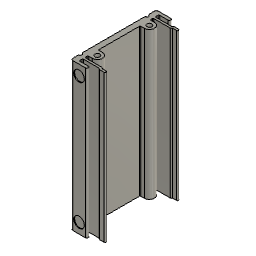
sidePanel_V2 v9 Fusion (Autodesk Fusion 360 design; units mm, degrees)
Autodesk Fusion 360 part; units mm, degrees
note: some values were not read from the file. Set by a fixed rule: which sketch regions a step uses.
sketch "Sketch1" plane through (0, 0, 0) normal (0, 0, 1) x (1, 0, 0)
  line L0 (36.0187, 148.7477) -> (36.0366, 148.794)
  line L1 (65.6521, 184) -> (76.1579, 184)
  line L2 (14.9996, 189) -> (14.9996, 194.9997)
  line L3 (-0.0194, 154.2247) -> (-0.0004, 154.2001)
  line L4 (-0.0302, 138.7537) -> (-0.0004, 138.7058)
  line L5 (-0.0004, 81.3672) -> (-0.0021, 81.3657)
  line L6 (15.3997, 143.0047) -> (15.3997, 102.5015)
  line L7 (-0.0004, 173.0047) -> (-0.0004, 102.5015)
  line L8 (2.0223, 183.0092) -> (1.9964, 183.0092)
  line L9 (1.9996, 175.0047) -> (2.0001, 175.0047)
  line L10 (4.0001, 177.0042) -> (4.0009, 181.0087)
  line L11 (0.0178, 200) -> (0.0178, 185.0092)
  arc A0 (0.0178, 185.0092) -> (2.0223, 183.0092) centre (2.0178, 185.0092) ccw
  arc A1 (4.0009, 181.0087) -> (1.9964, 183.0092) centre (2.0009, 181.0092) ccw
  line L12 (16.9996, 196.9997) -> (40, 196.9997)
  arc A2 (16.9996, 196.9997) -> (14.9996, 194.9997) centre (16.9996, 194.9997) ccw
  line L13 (16.9996, 187) -> (60, 187)
  arc A3 (14.9996, 189) -> (16.9996, 187) centre (16.9996, 189) ccw
  line L14 (63.5, 190) -> (76.1579, 190)
  line L15 (14.9996, 179.1547) -> (14.9996, 175.0047)
  arc A4 (16.9996, 181.1547) -> (14.9996, 179.1547) centre (16.9996, 179.1547) ccw
  line L16 (16.9996, 173.0047) -> (26.8487, 173.0047)
  arc A5 (14.9996, 175.0047) -> (16.9996, 173.0047) centre (16.9996, 175.0047) ccw
  arc A6 (2.0001, 175.0047) -> (4.0001, 177.0042) centre (2.0001, 177.0047) ccw
  arc A7 (1.9996, 175.0047) -> (-0.0004, 173.0047) centre (1.9996, 173.0047) ccw
  arc A8 (76.1579, 184) -> (76.1579, 190) centre (76.1579, 187) ccw
  line L17 (60, 187) -> (63.5, 190)
  line L18 (62.1079, 181.1547) -> (65.6521, 184)
  line L19 (17.3997, 145.0047) -> (27.1505, 145.0047)
  line L20 (27.4996, 145.0047) -> (27.5723, 145.0156)
  arc A9 (17.3997, 145.0047) -> (15.3997, 143.0047) centre (17.3997, 143.0047) ccw
  arc A10 (27.1505, 145.0047) -> (26.8487, 173.0047) centre (26.9996, 159.0047) ccw
  line L21 (-0.0004, 123.6359) -> (-0.0021, 123.6374)
  line L22 (5.0178, 205) -> (40, 205)
  arc A11 (5.0178, 205) -> (0.0178, 200) centre (5.0178, 200) ccw
  arc A12 (40, 196.9997) -> (40, 205) centre (40, 200.9999) ccw
  line L23 (16.9996, 181.1547) -> (62.1079, 181.1547)
  line L24 (27.4996, 29.9953) -> (27.5723, 29.9844)
  line L25 (16.9996, 1.9953) -> (26.8487, 1.9953)
  line L26 (16.9996, -12) -> (60, -12)
  line L27 (2.0223, -8.0092) -> (1.9964, -8.0092)
  line L28 (65.6521, -9) -> (76.1579, -9)
  arc A13 (1.9964, -8.0092) -> (4.0009, -6.0087) centre (2.0009, -6.0092) ccw
  line L29 (16.9996, -21.9997) -> (40, -21.9997)
  line L30 (1.9996, -0.0047) -> (2.0001, -0.0047)
  arc A14 (15.3997, 31.9953) -> (17.3997, 29.9953) centre (17.3997, 31.9953) ccw
  line L31 (36.0187, 26.2523) -> (36.0366, 26.206)
  arc A15 (0.0178, -25) -> (5.0178, -30) centre (5.0178, -25) ccw
  arc A16 (26.8487, 1.9953) -> (27.1505, 29.9953) centre (26.9996, 15.9953) ccw
  line L32 (4.0001, -2.0042) -> (4.0009, -6.0087)
  arc A17 (2.0223, -8.0092) -> (0.0178, -10.0092) centre (2.0178, -10.0092) ccw
  line L33 (16.9996, -6.1547) -> (62.1079, -6.1547)
  line L34 (5.0178, -30) -> (40, -30)
  arc A18 (16.9996, -12) -> (14.9996, -14) centre (16.9996, -14) ccw
  line L35 (14.9996, -4.1547) -> (14.9996, -0.0047)
  line L36 (63.5, -15) -> (76.1579, -15)
  arc A19 (40, -30) -> (40, -21.9997) centre (40, -25.9999) ccw
  arc A20 (76.1579, -15) -> (76.1579, -9) centre (76.1579, -12) ccw
  arc A21 (14.9996, -19.9997) -> (16.9996, -21.9997) centre (16.9996, -19.9997) ccw
  arc A22 (4.0001, -2.0042) -> (2.0001, -0.0047) centre (2.0001, -2.0047) ccw
  line L37 (-0.0004, 51.3641) -> (-0.0021, 51.3626)
  line L38 (17.3997, 29.9953) -> (27.1505, 29.9953)
  line L39 (60, -12) -> (63.5, -15)
  line L40 (-0.0004, 1.9953) -> (-0.0004, 72.4985)
  line L41 (0.0178, -25) -> (0.0178, -10.0092)
  line L42 (-0.0194, 20.7753) -> (-0.0004, 20.7999)
  line L43 (14.9996, -14) -> (14.9996, -19.9997)
  arc A23 (16.9996, 1.9953) -> (14.9996, -0.0047) centre (16.9996, -0.0047) ccw
  line L44 (62.1079, -6.1547) -> (65.6521, -9)
  line L45 (-0.0302, 36.2463) -> (-0.0004, 36.2942)
  arc A24 (-0.0004, 1.9953) -> (1.9996, -0.0047) centre (1.9996, 1.9953) ccw
  arc A25 (14.9996, -4.1547) -> (16.9996, -6.1547) centre (16.9996, -4.1547) ccw
  line L46 (15.3997, 31.9953) -> (15.3997, 72.4985)
  line L47 (-0.0004, 102.5015) -> (-0.0004, 72.4985)
  line L48 (15.3997, 102.5015) -> (15.3997, 72.4985)
  circle A26 centre (26.9996, 15.9953) radius 6.7755
  circle A27 centre (26.9996, 159.0047) radius 6.7755
  dimension "d8" = 2
  dimension "d9" = 2
  dimension "d11" = 2
  dimension "d13" = 2
  dimension "d18" = 2
  dimension "d19" = 2
  dimension "d27" = 2
  dimension "d28" = 2
  dimension "d34" = 3
  dimension "d35" = 2
  dimension "d40" = 5
  dimension "d41" = 4.0002
  dimension "d52" = 14.0008
  dimension "d55" = 235
  dimension "d57" = 14.0008
  dimension "d59" = 13.551
  dimension "d61" = 45.9953
  dimension "d62" = 45.9953
  dimension "d63" = 27
  dimension "d64" = 27
  dimension "d65" = 13.551
  constraint perpendicular L7 L9
  constraint tangent L11 A0
  constraint tangent L8 A0
  constraint tangent L8 A1
  constraint tangent L10 A1
  constraint horizontal L12
  constraint tangent L12 A2
  constraint tangent L2 A2
  constraint horizontal L13
  constraint tangent L2 A3
  constraint tangent L13 A3
  constraint horizontal L14
  constraint vertical L15
  constraint tangent L15 A4
  constraint horizontal L16
  constraint tangent L16 A5
  constraint tangent L15 A5
  constraint tangent L10 A6
  constraint tangent L9 A6
  constraint tangent L9 A7
  constraint tangent L7 A7
  constraint horizontal L1
  constraint tangent L14 A8
  constraint tangent L1 A8
  constraint horizontal L19
  constraint coincident L20.end A10
  constraint tangent L19 A9
  constraint tangent L6 A9
  constraint coincident L7 L3.end
  constraint coincident L7 L4.end
  constraint coincident L7 L5.start
  constraint vertical L7
  constraint vertical L6
  constraint horizontal L22
  constraint tangent L11 A11
  constraint tangent L22 A11
  constraint tangent L22 A12
  constraint tangent L12 A12
  constraint tangent A4 L23
  constraint horizontal L23
  constraint vertical L47
  constraint parallel L46 L48
  constraint concentric A16 A26
  constraint concentric A10 A27
  measures "d8" radius of A0
  measures "d9" radius of A1
  measures "d11" radius of A2
  measures "d13" radius of A3
  measures "d18" radius of A4
  measures "d19" radius of A5
  measures "d27" radius of A6
  measures "d28" radius of A7
  measures "d34" radius of A8
  measures "d35" radius of A9
  measures "d40" radius of A11
  measures "d41" radius of A12
  measures "d52" radius of A10
  measures "d55" distance of L22 L34
  measures "d57" radius of A16
  measures "d59" diameter of A26
  measures "d61" distance of A10.centre L22
  measures "d62" distance of A16.centre L34
  measures "d63" distance of L40 A16.centre
  measures "d64" distance of L7 A10.centre
  measures "d65" diameter of A27
extrude "Extrude4" add sketch "Sketch1" along normal blind 404.3634 contours L1 L2 L6 L7 L8 L10 L11 A0 A1 L12 A2 L13 A3 L14 L15 A4 L16 A5 A6 A7 A8 L17 L18 L19 A9 A10 L22 A11 A12 L23 L25 L26 L27 L28 A13 L29 A14 A15 A16 L32 A17 L33 L34 A18 L35 L36 A19 A20 A21 A22 L38 L39 L40 L41 L43 A23 L44 A24 A25 L46 L47 L48 | A26 | A27
sketch "Sketch2" plane through (0, 0, 404.3634) normal (0, 0, 1) x (-1, 0, 0)
  line L0 (-17.3997, -145.0047) -> (-27.1505, -145.0047)
  arc A0 (-27.1505, -145.0047) -> (-26.8487, -173.0047) centre (-26.9996, -159.0047) ccw
  line L1 (-26.8487, -173.0047) -> (-16.9996, -173.0047)
  arc A1 (-14.9996, -175.0047) -> (-16.9996, -173.0047) centre (-16.9996, -175.0047) ccw
  line L2 (-14.9996, -175.0047) -> (-14.9996, -179.1547)
  arc A2 (-16.9996, -181.1547) -> (-14.9996, -179.1547) centre (-16.9996, -179.1547) ccw
  line L3 (-16.9996, -181.1547) -> (-62.1079, -181.1547)
  line L4 (-62.1079, -181.1547) -> (-65.6521, -184)
  line L5 (-65.6521, -184) -> (-76.1579, -184)
  arc A3 (-76.1579, -184) -> (-76.1579, -190) centre (-76.1579, -187) ccw
  line L6 (-76.1579, -190) -> (-63.5, -190)
  line L7 (-63.5, -190) -> (-60, -187)
  line L8 (-60, -187) -> (-16.9996, -187)
  arc A4 (-14.9996, -189) -> (-16.9996, -187) centre (-16.9996, -189) ccw
  line L9 (-14.9996, -189) -> (-14.9996, -194.9997)
  arc A5 (-16.9996, -196.9997) -> (-14.9996, -194.9997) centre (-16.9996, -194.9997) ccw
  line L10 (-16.9996, -196.9997) -> (-40, -196.9997)
  arc A6 (-40, -196.9997) -> (-40, -205) centre (-40, -200.9999) ccw
  line L11 (-40, -205) -> (-5.0178, -205)
  arc A7 (-5.0178, -205) -> (-0.0178, -200) centre (-5.0178, -200) ccw
  line L12 (-0.0178, -200) -> (-0.0178, -185.0092)
  arc A8 (-0.0178, -185.0092) -> (-2.0223, -183.0092) centre (-2.0178, -185.0092) ccw
  line L13 (-2.0223, -183.0092) -> (-1.9964, -183.0092)
  arc A9 (-4.0009, -181.0087) -> (-1.9964, -183.0092) centre (-2.0009, -181.0092) ccw
  line L14 (-4.0009, -181.0087) -> (-4.0001, -177.0042)
  arc A10 (-2.0001, -175.0047) -> (-4.0001, -177.0042) centre (-2.0001, -177.0047) ccw
  line L15 (-2.0001, -175.0047) -> (-1.9996, -175.0047)
  arc A11 (-1.9996, -175.0047) -> (0.0004, -173.0047) centre (-1.9996, -173.0047) ccw
  line L16 (0.0004, -173.0047) -> (0.0004, -102.5015)
  line L17 (0.0004, -102.5015) -> (0.0004, -72.4985)
  line L18 (0.0004, -72.4985) -> (0.0004, -1.9953)
  arc A12 (0.0004, -1.9953) -> (-1.9996, 0.0047) centre (-1.9996, -1.9953) ccw
  line L19 (-1.9996, 0.0047) -> (-2.0001, 0.0047)
  arc A13 (-4.0001, 2.0042) -> (-2.0001, 0.0047) centre (-2.0001, 2.0047) ccw
  line L20 (-4.0001, 2.0042) -> (-4.0009, 6.0087)
  arc A14 (-1.9964, 8.0092) -> (-4.0009, 6.0087) centre (-2.0009, 6.0092) ccw
  line L21 (-1.9964, 8.0092) -> (-2.0223, 8.0092)
  arc A15 (-2.0223, 8.0092) -> (-0.0178, 10.0092) centre (-2.0178, 10.0092) ccw
  line L22 (-0.0178, 10.0092) -> (-0.0178, 25)
  arc A16 (-0.0178, 25) -> (-5.0178, 30) centre (-5.0178, 25) ccw
  line L23 (-5.0178, 30) -> (-40, 30)
  arc A17 (-40, 30) -> (-40, 21.9997) centre (-40, 25.9999) ccw
  line L24 (-40, 21.9997) -> (-16.9996, 21.9997)
  arc A18 (-14.9996, 19.9997) -> (-16.9996, 21.9997) centre (-16.9996, 19.9997) ccw
  line L25 (-14.9996, 19.9997) -> (-14.9996, 14)
  arc A19 (-16.9996, 12) -> (-14.9996, 14) centre (-16.9996, 14) ccw
  line L26 (-16.9996, 12) -> (-60, 12)
  line L27 (-60, 12) -> (-63.5, 15)
  line L28 (-63.5, 15) -> (-76.1579, 15)
  arc A20 (-76.1579, 15) -> (-76.1579, 9) centre (-76.1579, 12) ccw
  line L29 (-76.1579, 9) -> (-65.6521, 9)
  line L30 (-65.6521, 9) -> (-62.1079, 6.1547)
  line L31 (-62.1079, 6.1547) -> (-16.9996, 6.1547)
  arc A21 (-14.9996, 4.1547) -> (-16.9996, 6.1547) centre (-16.9996, 4.1547) ccw
  line L32 (-14.9996, 4.1547) -> (-14.9996, 0.0047)
  arc A22 (-16.9996, -1.9953) -> (-14.9996, 0.0047) centre (-16.9996, 0.0047) ccw
  line L33 (-16.9996, -1.9953) -> (-26.8487, -1.9953)
  arc A23 (-26.8487, -1.9953) -> (-27.1505, -29.9953) centre (-26.9996, -15.9953) ccw
  line L34 (-27.1505, -29.9953) -> (-17.3997, -29.9953)
  arc A24 (-15.3997, -31.9953) -> (-17.3997, -29.9953) centre (-17.3997, -31.9953) ccw
  line L35 (-15.3997, -31.9953) -> (-15.3997, -143.0047)
  arc A25 (-17.3997, -145.0047) -> (-15.3997, -143.0047) centre (-17.3997, -143.0047) ccw
  circle A26 centre (-26.9996, -15.9953) radius 6.7755
  circle A27 centre (-26.9996, -159.0047) radius 6.7755
  dimension "d66" = 13.551
  dimension "d67" = 13.551
  constraint concentric A23 A26
  constraint concentric A0 A27
  measures "d66" diameter of A26
  measures "d67" diameter of A27
hole "Hole1" at (26.9996, 159.0047, 404.3634) direction (0, 0, -1) diameter 13.551 end through all
sketch "Sketch3" plane through (0, 0, 404.3634) normal (0, 0, 1) x (-1, 0, 0)
  circle A0 centre (-26.9996, -159.0047) radius 6.7755
  line L0 (-17.3997, -145.0047) -> (-27.1505, -145.0047)
  arc A1 (-27.1505, -145.0047) -> (-26.8487, -173.0047) centre (-26.9996, -159.0047) ccw
  line L1 (-26.8487, -173.0047) -> (-16.9996, -173.0047)
  arc A2 (-14.9996, -175.0047) -> (-16.9996, -173.0047) centre (-16.9996, -175.0047) ccw
  line L2 (-14.9996, -175.0047) -> (-14.9996, -179.1547)
  arc A3 (-16.9996, -181.1547) -> (-14.9996, -179.1547) centre (-16.9996, -179.1547) ccw
  line L3 (-16.9996, -181.1547) -> (-62.1079, -181.1547)
  line L4 (-62.1079, -181.1547) -> (-65.6521, -184)
  line L5 (-65.6521, -184) -> (-76.1579, -184)
  arc A4 (-76.1579, -184) -> (-76.1579, -190) centre (-76.1579, -187) ccw
  line L6 (-76.1579, -190) -> (-63.5, -190)
  line L7 (-63.5, -190) -> (-60, -187)
  line L8 (-60, -187) -> (-16.9996, -187)
  arc A5 (-14.9996, -189) -> (-16.9996, -187) centre (-16.9996, -189) ccw
  line L9 (-14.9996, -189) -> (-14.9996, -194.9997)
  arc A6 (-16.9996, -196.9997) -> (-14.9996, -194.9997) centre (-16.9996, -194.9997) ccw
  line L10 (-16.9996, -196.9997) -> (-40, -196.9997)
  arc A7 (-40, -196.9997) -> (-40, -205) centre (-40, -200.9999) ccw
  line L11 (-40, -205) -> (-5.0178, -205)
  arc A8 (-5.0178, -205) -> (-0.0178, -200) centre (-5.0178, -200) ccw
  line L12 (-0.0178, -200) -> (-0.0178, -185.0092)
  arc A9 (-0.0178, -185.0092) -> (-2.0223, -183.0092) centre (-2.0178, -185.0092) ccw
  line L13 (-2.0223, -183.0092) -> (-1.9964, -183.0092)
  arc A10 (-4.0009, -181.0087) -> (-1.9964, -183.0092) centre (-2.0009, -181.0092) ccw
  line L14 (-4.0009, -181.0087) -> (-4.0001, -177.0042)
  arc A11 (-2.0001, -175.0047) -> (-4.0001, -177.0042) centre (-2.0001, -177.0047) ccw
  line L15 (-2.0001, -175.0047) -> (-1.9996, -175.0047)
  arc A12 (-1.9996, -175.0047) -> (0.0004, -173.0047) centre (-1.9996, -173.0047) ccw
  line L16 (0.0004, -173.0047) -> (0.0004, -102.5015)
  line L17 (0.0004, -102.5015) -> (0.0004, -72.4985)
  line L18 (0.0004, -72.4985) -> (0.0004, -1.9953)
  arc A13 (0.0004, -1.9953) -> (-1.9996, 0.0047) centre (-1.9996, -1.9953) ccw
  line L19 (-1.9996, 0.0047) -> (-2.0001, 0.0047)
  arc A14 (-4.0001, 2.0042) -> (-2.0001, 0.0047) centre (-2.0001, 2.0047) ccw
  line L20 (-4.0001, 2.0042) -> (-4.0009, 6.0087)
  arc A15 (-1.9964, 8.0092) -> (-4.0009, 6.0087) centre (-2.0009, 6.0092) ccw
  line L21 (-1.9964, 8.0092) -> (-2.0223, 8.0092)
  arc A16 (-2.0223, 8.0092) -> (-0.0178, 10.0092) centre (-2.0178, 10.0092) ccw
  line L22 (-0.0178, 10.0092) -> (-0.0178, 25)
  arc A17 (-0.0178, 25) -> (-5.0178, 30) centre (-5.0178, 25) ccw
  line L23 (-5.0178, 30) -> (-40, 30)
  arc A18 (-40, 30) -> (-40, 21.9997) centre (-40, 25.9999) ccw
  line L24 (-40, 21.9997) -> (-16.9996, 21.9997)
  arc A19 (-14.9996, 19.9997) -> (-16.9996, 21.9997) centre (-16.9996, 19.9997) ccw
  line L25 (-14.9996, 19.9997) -> (-14.9996, 14)
  arc A20 (-16.9996, 12) -> (-14.9996, 14) centre (-16.9996, 14) ccw
  line L26 (-16.9996, 12) -> (-60, 12)
  line L27 (-60, 12) -> (-63.5, 15)
  line L28 (-63.5, 15) -> (-76.1579, 15)
  arc A21 (-76.1579, 15) -> (-76.1579, 9) centre (-76.1579, 12) ccw
  line L29 (-76.1579, 9) -> (-65.6521, 9)
  line L30 (-65.6521, 9) -> (-62.1079, 6.1547)
  line L31 (-62.1079, 6.1547) -> (-16.9996, 6.1547)
  arc A22 (-14.9996, 4.1547) -> (-16.9996, 6.1547) centre (-16.9996, 4.1547) ccw
  line L32 (-14.9996, 4.1547) -> (-14.9996, 0.0047)
  arc A23 (-16.9996, -1.9953) -> (-14.9996, 0.0047) centre (-16.9996, 0.0047) ccw
  line L33 (-16.9996, -1.9953) -> (-26.8487, -1.9953)
  arc A24 (-26.8487, -1.9953) -> (-27.1505, -29.9953) centre (-26.9996, -15.9953) ccw
  line L34 (-27.1505, -29.9953) -> (-17.3997, -29.9953)
  arc A25 (-15.3997, -31.9953) -> (-17.3997, -29.9953) centre (-17.3997, -31.9953) ccw
  line L35 (-15.3997, -31.9953) -> (-15.3997, -143.0047)
  arc A26 (-17.3997, -145.0047) -> (-15.3997, -143.0047) centre (-17.3997, -143.0047) ccw
  circle A27 centre (-26.9996, -15.9953) radius 6.7755
  dimension "d70" = 13.551
  constraint concentric A24 A27
  measures "d70" diameter of A27
hole "Hole2" at (26.9996, 15.9953, 404.3634) direction (0, 0, -1) diameter 13.551 end through all
scale "Scale3" factor 0.21268 about (-0.0004, 102.5015, 0) bodies 1
sketch "Sketch4" plane through (0, 74.3211, 0) normal (0, -1, 0) x (1, 0, 0)
  line L0 (1.0669, 0) -> (8.5069, 0)
  line L1 (8.5069, 0) -> (8.5069, 86)
  line L2 (8.5069, 86) -> (1.0669, 86)
  line L3 (1.0669, 86) -> (1.0669, 0)
  circle A0 centre (4.7869, 80) radius 3.1
  circle A1 centre (4.7869, 6) radius 3.1
  dimension "d73" = 6.2
  dimension "d74" = 7.44
  dimension "d75" = 3.72
  dimension "d76" = 6
  dimension "d77" = 6.2
  dimension "d78" = 3.72
  dimension "d79" = 6
  measures "d73" diameter of A0
  measures "d74" distance of L1.end L2.end
  measures "d75" distance of L3 A0.centre
  measures "d76" distance of L2 A0.centre
  measures "d77" diameter of A1
  measures "d78" distance of L3 A1.centre
  measures "d79" distance of L0 A1.centre
extrude "Extrude5" cut sketch "Sketch4" against normal blind 0.5 contours A0 | A1
